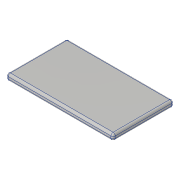
# Autodesk Inventor part: battery
Saved by Autodesk Inventor 2017 (Build 210142000, 142)
## iProperties
Created: 2016-08-01
Part Number: battery
Material: Generic
Document SubType Name: Modeling
Designer: ge937963
Density: 1 g/cm^3
Appearance: Aluminum - Flat
Mass: 6.29263 g
Surface Area: 31.9999 cm^2
Volume: 6.29263 cm^3
Author: ge937963
Autodesk Inventor part; units mm, degrees
ref_plane "YZ Plane" through (0, 0, 0) normal (1, 0, 0) x (0, 1, 0)
ref_plane "XZ Plane" through (0, 0, 0) normal (0, 1, 0) x (-1, 0, 0)
ref_plane "XY Plane" through (0, 0, 0) normal (0, 0, 1) x (1, 0, 0)
sketch "Sketch1" plane through (0, 0, 0) normal (0, 1, 0) x (-1, 0, 0)
  line L0 (0, 0) -> (63.5, 0)
  line L1 (63.5, 0) -> (63.5, -36.068)
  line L2 (63.5, -36.068) -> (0, -36.068)
  line L3 (0, -36.068) -> (0, 0)
  dimension "d0" = 63.5
  dimension "d1" = 36.068
  constraints: 8 end point, 2 parallel, 1 horizontal, 1 perpendicular
  measures "d0" distance of L1.end L2.end
  measures "d1" distance of L0.end L1.end
extrude "Extrusion1" add sketch "Sketch1" along normal blind 3.81
sketch "Sketch2" plane through (0, 0, 0) normal (1, 0, 0) x (0, 0, -1)
  point P0 (0, 0)
fillet "Fillet1" radius 1.27 12 edges at (-31.75, 3.81, 0) (-31.75, 3.81, -36.068) (-31.75, 0, 0) (-31.75, 0, -36.068) (0, 0, -18.034) (0, 3.81, -18.034) (0, 1.905, 0) (0, 1.905, -36.068) (-63.5, 1.905, -36.068) (-63.5, 3.81, -18.034) (-63.5, 1.905, 0) (-63.5, 0, -18.034)
body "Solid1"
